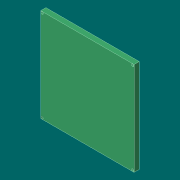
# Autodesk Inventor part: front
Saved by Autodesk Inventor 2016 (Build 200138000, 138)
## iProperties
Created: 2015-10-13
Part Number: front
Material: PC/ABS Plastic
Document SubType Name: Modeling
Designer: Sawaiz
Density: 0.357273 g/cm^3
Appearance: Smooth - Dark Sea Green
Author: Sawaiz
Autodesk Inventor part; units mm, degrees
ref_plane "YZ Plane" through (0, 0, 0) normal (1, 0, 0) x (0, 1, 0)
ref_plane "XZ Plane" through (0, 0, 0) normal (0, 1, 0) x (-1, 0, 0)
ref_plane "XY Plane" through (0, 0, 0) normal (0, 0, 1) x (1, 0, 0)
sketch "Sketch1" plane through (0, 0, 0) normal (1, 0, 0) x (0, 1, 0)
  line L0 (-57.15, -57.15) -> (57.15, -57.15)
  line L1 (57.15, -57.15) -> (57.15, 57.15)
  line L2 (57.15, 57.15) -> (-57.15, 57.15)
  line L3 (-57.15, 57.15) -> (-57.15, -57.15)
  line L4 (-57.15, -57.15) -> (57.15, 57.15) construction
  line L5 (57.15, -57.15) -> (-57.15, 57.15) construction
  point P0 (0, 0)
  dimension "d0" = 114.3
  dimension "d1" = 114.3
  constraints: 12 end point, 2 midpoint, 2 parallel, 1 horizontal, 1 perpendicular
  measures "d0" distance of L2.end L1.end
  measures "d1" distance of L1.end L0.end
extrude "Extrusion1" add sketch "Sketch1" along normal blind 6.35
sketch "Sketch2" plane through (6.35, 0, 0) normal (1, 0, 0) x (0, 0, -1)
  line L0 (57.15, -57.15) -> (57.15, 57.15) projected
  line L1 (57.15, 57.15) -> (-57.15, 57.15) projected
  line L2 (-57.15, 57.15) -> (-57.15, -57.15) projected
  line L3 (-57.15, -57.15) -> (57.15, -57.15) projected
  line L4 (-55.5625, -57.15) -> (-55.5625, 57.15)
  point P0 (0, 0)
  point P1 (-55.5625, -55.5625)
  point P2 (-55.5625, 55.5625)
  dimension "d4" = 1.5875
  dimension "d29" = 1.5875
  dimension "d30" = 1.5875
  constraints: 4 point on line, 2 end point, 1 vertical
  measures "d4" distance between parallel lines of L2 L4
  measures "d29" distance from line of L3 point (-55.562, -55.562)
  measures "d30" distance from line of L1 point (-55.562, 55.563)
hole "Hole1" at (6.35, -55.5625, 55.5625) at (6.35, 55.5625, 55.5625) direction (-1, 0, 0) diameter 1.778 end through all countersink diameter 3.023 countersink angle 82 clearance for "Flat Head Machine Screw (82)" size "#0" standard "Ansi Unified Screw Threads"
mirror "Mirror1" about plane through (0, 0, 0) normal (0, 0, 1) of "Hole1"
sketch "Sketch4" plane through (0, 0, 0) normal (-1, 0, 0) x (0, 0, 1)
  line L0 (-52.3875, 52.3875) -> (52.3875, 52.3875)
  line L1 (52.3875, 52.3875) -> (52.3875, -52.3875)
  line L2 (52.3875, -52.3875) -> (-52.3875, -52.3875)
  line L3 (-52.3875, -52.3875) -> (-52.3875, 52.3875)
  line L4 (-52.3875, 52.3875) -> (52.3875, -52.3875) construction
  line L5 (52.3875, 52.3875) -> (-52.3875, -52.3875) construction
  line L6 (55.5625, -52.3875) -> (55.5625, 52.3875)
  line L7 (52.3875, 55.5625) -> (-52.3875, 55.5625)
  line L8 (-55.5625, 52.3875) -> (-55.5625, -52.3875)
  line L9 (-52.3875, -55.5625) -> (52.3875, -55.5625)
  arc A0 (55.5625, 52.3875) -> (52.3875, 55.5625) centre (52.3875, 52.3875) ccw
  arc A1 (52.3875, -55.5625) -> (55.5625, -52.3875) centre (52.3875, -52.3875) ccw
  arc A2 (-55.5625, -52.3875) -> (-52.3875, -55.5625) centre (-52.3875, -52.3875) ccw
  arc A3 (-52.3875, 55.5625) -> (-55.5625, 52.3875) centre (-52.3875, 52.3875) ccw
  point P0 (0, 0)
  dimension "d27" = 104.775
  dimension "d28" = 104.775
  dimension "d31" = 3.175
  dimension "d32" = 3.175
  constraints: 20 end point, 8 point on circle, 8 tangent, 4 centre point, 4 parallel, 3 equal radius, 2 midpoint, 2 perpendicular, 1 horizontal, 3 other
  measures "d27" distance of L1.end L2.end
  measures "d28" distance of L0.end L1.end
  measures "d31" distance between parallel lines of L1 L6
  measures "d32" radius of A0
extrude "Extrusion2" cut sketch "Sketch4" against normal blind 0.9525
equation "\"d0\" = width + 2 * acrylicThickness"
equation "\"d1\" = height + 2 * acrylicThickness"
equation "\"d2\" = acrylicThickness"
equation "\"d4\" = 0.25 * acrylicThickness"
equation "\"d29\" = 0.25 * acrylicThickness"
equation "\"d30\" = 0.25 * acrylicThickness"
equation "\"d27\" = 0.25 * frontBackORingID"
equation "\"d28\" = 0.25 * frontBackORingID"
equation "\"d31\" = oRingWidth"
equation "\"d32\" = oRingWidth"
equation "\"acrylicThickness\" = 6.35"
equation "\"height\" = 101.6"
equation "\"width\" = 101.6"
equation "\"depth\" = 101.6"
equation "\"mirrorAngle\" = 5deg"
equation "\"detectorWidth\" = 52"
equation "\"detectorHeight\" = 52"
equation "\"mirrorThickness\" = 3"
equation "\"fresnelThickness\" = 0.1"
equation "\"ior\" = 1.49"
equation "\"focalLength\" = 76.2"
equation "\"fresnelAngle\" = 90deg"
equation "\"centerThickness\" = 1.524"
equation "\"fresnelEffectiveDiameter\" = 76.2"
equation "\"mirrorSuppourtWidth\" = 38.1"
equation "\"backGrooveBit\" = 4.8006"
equation "\"sensorHolderSensorWidth\" = 53.975"
equation "\"sensorHolderHeight\" = 88.9"
equation "\"sensorHolderSesnorHeight\" = 53.975"
equation "\"sensorHolderWidth\" = 88.9"
equation "\"sensorHolderSensorHeight\" = 53.975"
equation "\"sensorHolderORingGroove\" = 3.175"
equation "\"sensorHolderORing\" = 3.175"
equation "\"sensorHolderFlushORing\" = 3.175"
equation "\"sensorHolderFlushORingID\" = 304.8"
equation "\"frontBackORingID\" = 419.1"
equation "\"sensorHolderORingID\" = 203.2"
equation "\"oRingWidth\" = 3.175"
equation "\"topBottomHorizontalMirrorGroove\" = 12.7"
equation "\"backMirrorGroove\" = 6.35"
equation "\"mirrorGroove\" = 19.05"
equation "\"fresnelChamfer\" = 6.35"
equation "\"mirrorGrooveFillet\" = 6.35"
equation "\"mirrorGrooveDrill\" = 6.35"
equation "\"mirrorGrooveMill\" = 3.175"
equation "\"fresnelMirrorChamfer\" = 6.35"
equation "\"detectorOpeningHeight\" = 76.2"
equation "\"detectorOpeningWidth\" = 76.2"
body "Solid1"
